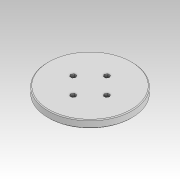
# Autodesk Inventor part: Platform
Saved by Autodesk Inventor 2020 (Build 240168000, 168)
## iProperties
Created: 2021-08-24
Part Number: Platform
Material: Generic
Document SubType Name: Modeling
Designer: DDeGo
Density: 1 g/cm^3
Appearance: Default
Author: DDeGo
Autodesk Inventor part; units mm, degrees
ref_plane "YZ Plane" through (0, 0, 0) normal (1, 0, 0) x (0, 1, 0)
ref_plane "XZ Plane" through (0, 0, 0) normal (0, 1, 0) x (-1, 0, 0)
ref_plane "XY Plane" through (0, 0, 0) normal (0, 0, 1) x (1, 0, 0)
sketch "Sketch1" plane through (0, 0, 0) normal (0, 0, 1) x (1, 0, 0)
  line L0 (0, 0) -> (16.5, 0) construction
  line L1 (16.5, 0) -> (16.5, 7)
  line L2 (16.5, 7) -> (0, 7)
  line L3 (0, 7) -> (0, 9)
  line L4 (0, 9) -> (50, 9)
  line L5 (50, 9) -> (50, 0)
  line L6 (50, 0) -> (16.5, 0)
  line L7 (0, 7) -> (0, 0) construction
  dimension "d0" = 16.5
  dimension "d1" = 7
  dimension "d2" = 2
  dimension "d3" = 50
  constraints: 16 end point, 6 perpendicular, 1 horizontal, 1 point on line, 1 vertical
  measures "d0" distance between parallel lines of L1 L7
  measures "d1" distance of L0.end L1.end
  measures "d2" distance between parallel lines of L2 L4
  measures "d3" distance between parallel lines of L3 L5
revolve "Revolution1" add sketch "Sketch1" angle 360 about axis through (0, 7, 0) along (0, 1, 0)
sketch "Sketch2" plane through (0, 0, 0) normal (0, -1, 0) x (1, 0, 0)
  line L0 (0, 20) -> (0, -20) construction
  line L1 (-4.2, 20) -> (-4.2, -20)
  line L2 (4.2, -20) -> (4.2, 20)
  arc A0 (4.2, 20) -> (-4.2, 20) centre (0, 20) ccw
  arc A1 (-4.2, -20) -> (4.2, -20) centre (0, -20) ccw
  line L3 (-20, 0) -> (20, 0) construction
  line L4 (-20, -4.2) -> (20, -4.2)
  line L5 (20, 4.2) -> (-20, 4.2)
  arc A2 (-20, 4.2) -> (-20, -4.2) centre (-20, 0) ccw
  arc A3 (20, -4.2) -> (20, 4.2) centre (20, 0) ccw
  point P0 (0, 0)
  point P1 (4.2, 4.2)
  point P2 (-4.2, 4.2)
  point P3 (-4.2, -4.2)
  point P4 (4.2, -4.2)
  dimension "d5" = 4.2
  dimension "d6" = 40
  dimension "d7" = 40
  constraints: 16 end point, 8 point on circle, 8 tangent, 4 centre point, 2 midpoint, 2 parallel, 1 equal radius, 1 perpendicular, 1 vertical
  measures "d5" radius of A3
  measures "d6" distance of L0.start L0.end
  measures "d7" distance of L3.start L3.end
extrude "Extrusion1" cut sketch "Sketch2" against normal blind 1.5
sketch "Sketch3" plane through (0, 1.5, 0) normal (0, -1, 0) x (1, 0, 0)
  arc A0 (4.2, 20) -> (-4.2, 20) centre (0, 20) ccw projected
  circle A1 centre (0, 20) radius 1.7
  arc A2 (20, -4.2) -> (20, 4.2) centre (20, 0) ccw projected
  circle A3 centre (20, 0) radius 1.7
  arc A4 (-4.2, -20) -> (4.2, -20) centre (0, -20) ccw projected
  circle A5 centre (0, -20) radius 1.7
  arc A6 (-20, 4.2) -> (-20, -4.2) centre (-20, 0) ccw projected
  circle A7 centre (-20, 0) radius 1.7
  point P0 (0, 0)
  dimension "d10" = 3.4
  constraints: 4 centre point, 4 coincident, 3 equal radius
  measures "d10" diameter of A3
extrude "Extrusion2" cut sketch "Sketch3" against normal through all
sketch "Sketch4" plane through (0, 9, 0) normal (0, 1, 0) x (1, 0, 0)
  circle A0 centre (0, -20) radius 1.7 projected
  line L0 (-1.6454, -17.15) -> (1.6454, -17.15)
  line L1 (1.6454, -17.15) -> (3.2909, -20)
  line L2 (3.2909, -20) -> (1.6454, -22.85)
  line L3 (1.6454, -22.85) -> (-1.6454, -22.85)
  line L4 (-1.6454, -22.85) -> (-3.2909, -20)
  line L5 (-3.2909, -20) -> (-1.6454, -17.15)
  circle A1 centre (0, 20) radius 1.7 projected
  line L6 (-1.6454, 17.15) -> (-3.2909, 20)
  line L7 (-3.2909, 20) -> (-1.6454, 22.85)
  line L8 (-1.6454, 22.85) -> (1.6454, 22.85)
  line L9 (1.6454, 22.85) -> (3.2909, 20)
  line L10 (3.2909, 20) -> (1.6454, 17.15)
  line L11 (1.6454, 17.15) -> (-1.6454, 17.15)
  circle A2 centre (20, 0) radius 1.7 projected
  line L12 (21.6454, 2.85) -> (23.2909, 0)
  line L13 (23.2909, 0) -> (21.6454, -2.85)
  line L14 (21.6454, -2.85) -> (18.3546, -2.85)
  line L15 (18.3546, -2.85) -> (16.7091, 0)
  line L16 (16.7091, 0) -> (18.3546, 2.85)
  line L17 (18.3546, 2.85) -> (21.6454, 2.85)
  circle A3 centre (-20, 0) radius 1.7 projected
  line L18 (-21.6454, 2.85) -> (-18.3546, 2.85)
  line L19 (-18.3546, 2.85) -> (-16.7091, 0)
  line L20 (-16.7091, 0) -> (-18.3546, -2.85)
  line L21 (-18.3546, -2.85) -> (-21.6454, -2.85)
  line L22 (-21.6454, -2.85) -> (-23.2909, 0)
  line L23 (-23.2909, 0) -> (-21.6454, 2.85)
  point P0 (0, 0)
  point P1 (0, -20)
  point P2 (0, 20)
  dimension "d13" = 5.7
  constraints: 48 end point, 4 coincident, 4 horizontal, 3 equal length, 52 other
  measures "d13" distance between parallel lines of L19 L22
extrude "Extrusion3" cut sketch "Sketch4" against normal blind 3.5 contours A0 | L0 L1 L2 L3 L4 L5 | A1 | L6 L7 L8 L9 L10 L11 | A2 | L12 L13 L14 L15 L16 L17 | A3 | L18 L19 L20 L21 L22 L23
chamfer "Chamfer1" distance 1 angle 45 2 edges at (-50, 0, 0) (-50, 9, 0)
chamfer "Chamfer2" distance 1 angle 45 4 edges at (-11.6673, 0, -11.6673) (-11.6673, 0, 11.6673) (11.6673, 0, 11.6673) (11.6673, 0, -11.6673)
body "Solid1"
